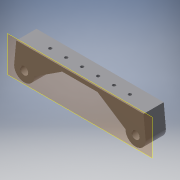
# Autodesk Inventor part: Bed
Saved by Autodesk Inventor 2016 (Build 200138000, 138)
## iProperties
Created: 2016-04-23
Part Number: Bed
Material: Generic
Document SubType Name: Modeling
Designer: Scott
Density: 1 g/cm^3
Appearance: Default
Author: Scott
Autodesk Inventor part; units mm, degrees
ref_plane "YZ Plane" through (0, 0, 0) normal (1, 0, 0) x (0, 1, 0)
ref_plane "XZ Plane" through (0, 0, 0) normal (0, 1, 0) x (-1, 0, 0)
ref_plane "XY Plane" through (0, 0, 0) normal (0, 0, 1) x (1, 0, 0)
ref_plane "Work Plane1" through (0, 0, 0) normal (0, 0, 1) x (1, 0, 0)
sketch "Sketch1" plane through (0, 0, 0) normal (0, 0, 1) x (1, 0, 0)
  circle A0 centre (-70.0994, -13.8265) radius 7.5 projected
  circle A1 centre (69.9006, -13.8265) radius 7.5 projected
  circle A2 centre (-0.0994, -13.8265) radius 5.08 projected
  arc A3 (-82.5729, -11.3834) -> (-57.3889, -13.8265) centre (-70.0994, -13.8265) ccw projected
  line L0 (-57.3889, 5.8585) -> (-57.3889, -13.8265) projected
  line L1 (-54.2139, 9.0335) -> (-57.3889, 5.8585) projected
  line L2 (-25.4994, 9.0335) -> (-54.2139, 9.0335) projected
  arc A4 (-17.8794, 1.4135) -> (-25.4994, 9.0335) centre (-25.4994, 1.4135) ccw projected
  line L3 (-17.8794, -26.5265) -> (-17.8794, 1.4135) projected
  line L4 (17.6806, -26.5265) -> (-17.8794, -26.5265) projected
  line L5 (17.6806, 1.4135) -> (17.6806, -26.5265) projected
  arc A5 (25.3006, 9.0335) -> (17.6806, 1.4135) centre (25.3006, 1.4135) ccw projected
  line L6 (54.0151, 9.0335) -> (25.3006, 9.0335) projected
  line L7 (57.1901, 5.8585) -> (54.0151, 9.0335) projected
  line L8 (57.1901, -13.8265) -> (57.1901, 5.8585) projected
  arc A6 (57.1901, -13.8265) -> (82.6111, -13.8265) centre (69.9006, -13.8265) ccw projected
  line L9 (79.9006, 14.1135) -> (82.6111, -13.8265) projected
  line L10 (-80.0994, 14.1135) -> (79.9006, 14.1135) projected
  line L11 (-82.5729, -11.3834) -> (-80.0994, 14.1135) projected
  line L12 (-25.4994, 9.0335) -> (25.3006, 9.0335)
  point P0 (0, 0)
  constraints: 2 end point, 1 horizontal, 1 point on circle
extrude "Extrusion1" add sketch "Sketch1" against normal blind 25.4 contours L11 L10 L9 A6 L8 L7 L6 L12 L2 L1 L0 A3
sketch "Sketch2" plane through (0, 0, 0) normal (0, 0, 1) x (1, 0, 0)
  circle A0 centre (69.9006, -13.8265) radius 7.5 projected
  circle A1 centre (-70.0994, -13.8265) radius 7.5 projected
  line L0 (-57.3889, -13.8265) -> (-57.3889, 5.8585) projected
  line L1 (-57.3889, 5.8585) -> (-54.2139, 9.0335) projected
  line L2 (-54.2139, 9.0335) -> (54.0151, 9.0335) projected
  line L3 (54.0151, 9.0335) -> (57.1901, 5.8585) projected
  line L4 (57.1901, 5.8585) -> (57.1901, -13.8265) projected
  arc A2 (57.1901, -13.8265) -> (82.6111, -13.8265) centre (69.9006, -13.8265) ccw projected
  line L5 (82.6111, -13.8265) -> (79.9006, 14.1135) projected
  line L6 (79.9006, 14.1135) -> (-80.0994, 14.1135) projected
  line L7 (-80.0994, 14.1135) -> (-82.5729, -11.3834) projected
  arc A3 (-82.5729, -11.3834) -> (-57.3889, -13.8265) centre (-70.0994, -13.8265) ccw projected
  circle A4 centre (-70.0994, -13.8265) radius 5
  circle A5 centre (69.9006, -13.8265) radius 5
  point P0 (0, 0)
  dimension "d2" = 10
  dimension "d3" = 10
  constraints: 2 centre point, 2 coincident
  measures "d2" diameter of A4
  measures "d3" diameter of A5
extrude "Extrusion2" add sketch "Sketch2" against normal blind 1 contours A0 | A1
sketch "Sketch3" plane through (-54.2139, 9.0335, 0) normal (0, -1, 0) x (1, 0, 0)
  line L0 (0, 0) -> (108.229, 0) projected
  line L1 (108.229, -25.4) -> (0, -25.4) projected
  line L2 (-11.8855, 142.225) -> (-11.8855, -175.0375)
  line L3 (-25.8855, -146.05) -> (-25.8855, 93.95) projected
  line L4 (-25.8855, 0) -> (-25.8855, -25.4) projected
  line L5 (-25.8855, -12.7) -> (4.1145, -12.7)
  circle A0 centre (4.1145, -12.7) radius 2
  circle A1 centre (24.1145, -12.7) radius 2
  circle A2 centre (44.1145, -12.7) radius 2
  line L6 (54.2139, 0) -> (54.2139, -3.82)
  line L7 (134.3133, -12.7) -> (104.3133, -12.7)
  circle A3 centre (104.3133, -12.7) radius 2
  circle A4 centre (84.3133, -12.7) radius 2
  circle A5 centre (64.3133, -12.7) radius 2
  dimension "d6" = 30
  dimension "d9" = 4
  dimension "d10" = 4
  dimension "d11" = 4
  constraints: 8 end point, 6 centre point, 5 symmetric about line, 2 coincident, 2 vertical, 1 horizontal, 1 midpoint, 5 other
  measures "d6" distance of L5.start L5.end
  measures "d9" diameter of A0
  measures "d10" diameter of A1
  measures "d11" diameter of A2
extrude "Extrusion3" cut sketch "Sketch3" against normal blind 508
sketch "Sketch4" plane through (0, 0, 0) normal (0, 0, 1) x (1, 0, 0)
  circle A0 centre (69.9006, -13.8265) radius 5 projected
  circle A1 centre (-70.0994, -13.8265) radius 5 projected
  line L0 (-57.3889, -13.8265) -> (-57.3889, 5.8585) projected
  line L1 (-57.3889, 5.8585) -> (-54.2139, 9.0335) projected
  line L2 (-54.2139, 9.0335) -> (54.0151, 9.0335) projected
  line L3 (54.0151, 9.0335) -> (57.1901, 5.8585) projected
  line L4 (57.1901, 5.8585) -> (57.1901, -13.8265) projected
  arc A2 (57.1901, -13.8265) -> (82.6111, -13.8265) centre (69.9006, -13.8265) ccw projected
  line L5 (82.6111, -13.8265) -> (79.9006, 14.1135) projected
  line L6 (79.9006, 14.1135) -> (-80.0994, 14.1135) projected
  line L7 (-80.0994, 14.1135) -> (-82.5729, -11.3834) projected
  arc A3 (-82.5729, -11.3834) -> (-57.3889, -13.8265) centre (-70.0994, -13.8265) ccw projected
  line L8 (-57.3889, -13.8265) -> (-22.2837, 9.0335)
  line L9 (54.0151, 9.0335) -> (-54.2139, 9.0335) projected
  line L10 (-0.0994, 9.0335) -> (-0.0994, 6.3526)
  line L11 (-57.3889, 5.8585) -> (-57.3889, -13.8265) projected
  line L12 (-57.3889, -13.8265) -> (-57.3889, 9.0335)
  line L13 (-57.3889, 9.0335) -> (-22.2837, 9.0335)
  line L14 (57.1901, -13.8265) -> (57.1901, 5.8585)
  line L15 (54.0151, 9.0335) -> (-54.2139, 9.0335)
  line L16 (57.1901, -13.8265) -> (22.0849, 9.0335)
  line L17 (57.1901, -13.8265) -> (57.1901, 9.0335)
  line L18 (57.1901, 9.0335) -> (22.0849, 9.0335)
  point P0 (0, 0)
  constraints: 18 end point, 4 symmetric about line, 1 midpoint, 1 perpendicular, 1 point on line, 1 vertical
extrude "Extrusion4" add sketch "Sketch4" against normal blind 5.08 contours L0 L1 L2 L8 | L2 L3 L4 L16 | L18 L17 L3
body "Solid1"
